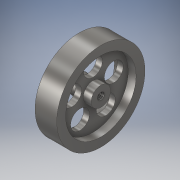
# Autodesk Inventor part: fly wheel
Saved by Autodesk Inventor 2018 (Build 220112000, 112)
## iProperties
Created: 2018-02-14
Part Number: fly wheel
Material: Iron, Malleable
Document SubType Name: Modeling
Designer: 238438
Density: 7.15 g/cm^3
Appearance: Semi-Polished
Mass: 15.6592 g
Surface Area: 22.6756 cm^2
Volume: 2.1901 cm^3
Author: 238438
Autodesk Inventor part; units mm, degrees
ref_plane "YZ Plane" through (0, 0, 0) normal (1, 0, 0) x (0, 1, 0)
ref_plane "XZ Plane" through (0, 0, 0) normal (0, 1, 0) x (-1, 0, 0)
ref_plane "XY Plane" through (0, 0, 0) normal (0, 0, 1) x (1, 0, 0)
sketch "Sketch3" plane through (0, 0, 0) normal (0, 1, 0) x (-1, 0, 0)
  line L0 (68.9195, -10.287) -> (-79.2178, -10.287)
  line L1 (-11.0342, -11.43) -> (-17.9938, -11.43)
  line L2 (-17.9938, -11.43) -> (-17.9938, -13.3858)
  line L3 (-11.0342, -11.43) -> (-11.0342, -13.3858)
  line L4 (-11.0342, -13.3858) -> (-13.5742, -13.3858)
  line L5 (-17.9938, -13.3858) -> (-15.4538, -13.3858)
  line L6 (-15.4538, -13.3858) -> (-15.4538, -21.59)
  line L7 (-13.5742, -13.3858) -> (-13.5742, -21.59)
  line L8 (-13.5742, -21.59) -> (-11.0342, -21.59)
  line L9 (-15.4538, -21.59) -> (-17.9938, -21.59)
  line L10 (-17.9938, -21.59) -> (-17.9938, -24.4348)
  line L11 (-11.0342, -21.59) -> (-11.0342, -24.4348)
  line L12 (-11.0342, -24.4348) -> (-17.9938, -24.4348)
  point P0 (0, 0)
  dimension "d10" = 1.143
  dimension "d11" = 6.9596
  dimension "d12" = 1.9558
  dimension "d13" = 2.54
  dimension "d14" = 2.54
  dimension "d15" = 8.2042
  dimension "d16" = 2.8448
  constraints: 26 end point, 5 perpendicular, 4 horizontal, 4 vertical
  measures "d10" distance between parallel lines of L0 L1
  measures "d11" distance of L1.end L1.start
  measures "d12" distance of L1.end L2.end
  measures "d13" distance of L3.end L4.end
  measures "d14" distance of L2.end L5.end
  measures "d15" distance of L5.end L6.end
  measures "d16" distance of L9.end L10.end
revolve "Revolution1" add sketch "Sketch3" angle 360 about axis through (-68.9195, 0, -10.287) along (1, 0, 0)
thread "Thread1" size "3-48 UNC" class "2B" standard "ANSI Unified Screw Threads" full length
sketch "Sketch4" plane through (15.4538, 0, -10.287) normal (1, 0, 0) x (0, 0, -1)
  circle A0 centre (0.0087, 7.0124) radius 3.0353
  circle A1 centre (-6.6665, 2.1752) radius 3.0353
  circle A2 centre (-4.1289, -5.6681) radius 3.0353
  circle A3 centre (4.1148, -5.6783) radius 3.0353
  circle A4 centre (6.6719, 2.1587) radius 3.0353
  point P0 (-10.287, 0)
  point P1 (0, 0)
  dimension "d20" = 6.0706
  dimension "d23" = 360
  constraints: 5 centre point, 11 other
  measures "d20" diameter of A0
extrude "Extrusion3" cut sketch "Sketch4" against normal through all
body "Solid2"
